dewalt_gyro_screwdriver_holder_v4 (Autodesk Fusion 360 design; units mm, degrees)
Autodesk Fusion 360 part; units mm, degrees
sketch "Sketch1" plane through (0, 0, 0) normal (0, 0, 1) x (1, 0, 0)
  line L0 (0, 0) -> (38.1, 0)
  line L1 (38.1, 0) -> (38.1, 38.1)
  line L2 (38.1, 38.1) -> (0, 38.1)
  line L3 (0, 38.1) -> (0, 0)
  dimension "d1" = 38.1
  dimension "d2" = 38.1
  constraint horizontal L0
  constraint vertical L1
  constraint horizontal L2
  constraint vertical L3
  constraint coincident L0.start L3.end
  measures "d1" distance of L0.start L2.end
  measures "d2" distance of L0.start L0.end
extrude "Extrude1" add sketch "Sketch1" along normal blind 1 makes body 1
sketch "Sketch3" plane through (0, 38.1, 0) normal (0, 1, 0) x (-1, 0, 0)
  line L0 (-38.1, 0) -> (0, 0)
  line L1 (0, 0) -> (0, 1)
  line L2 (0, 1) -> (-38.1, 1)
  line L3 (-38.1, 1) -> (-38.1, 0)
  circle A0 centre (-19.05, 13) radius 10
  line L4 (-7.05, 1) -> (-31.05, 1)
  line L5 (-31.05, 1) -> (-31.05, 13)
  line L6 (-19.05, 25) -> (-19.05, 25)
  line L7 (-7.05, 13) -> (-7.05, 1)
  arc A1 (-7.05, 13) -> (-19.05, 25) centre (-19.05, 13) ccw
  arc A2 (-19.05, 25) -> (-31.05, 13) centre (-19.05, 13) ccw
  dimension "d40" = 20
  dimension "d44" = 12
  dimension "d45" = 12
  dimension "d46" = 12
  dimension "d48" = 19.05
  dimension "d49" = 19.05
  dimension "d50" = 12
  constraint horizontal L4
  constraint vertical L5
  constraint vertical L7
  constraint coincident L2 L4.start
  constraint tangent L7 A1
  constraint tangent L5 A2
  constraint equal A1 A2
  measures "d40" diameter of A0
  measures "d44" distance of L2 A0.centre
  measures "d45" distance of A0.centre L7
  measures "d46" distance of A0.centre L5
  measures "d48" distance of L3 A0.centre
  measures "d49" distance of L1 A0.centre
  measures "d50" radius of A1
extrude "Extrude9" add sketch "Sketch3" against normal blind 46 separate body contours A0 makes body 2
extrude "Extrude2" add sketch "Sketch3" along normal blind 20 separate body contours L2 L4 L5 L7 A1 A2 | A0 makes body 3
move_body "Move1" bodies 3 to x (1, 0, 0) y (0, 1, 0) z (0, 0, 1) at (0, -32, 0)
move_body "Align1" bodies 3 to x (1, 0, 0) y (0, 1, 0) z (0, 0, 1) at (-0.0025, 2.95, -24)
move_body "Move2" bodies 3 to x (1, 0, 0) y (0, 1, 0) z (0, 0, 1) at (0, 0, 27)
move_body "Move3" bodies 3 to x (1, 0, 0) y (0, 1, 0) z (0, 0, 1) at (0, 0, 5)
move_body "Align2" bodies 3 to x (1, 0, 0) y (0, 1, 0) z (0, 0, 1) at (0, 0, -8)
fillet "Fillet1" radius 6 1 edges at (38.1, 38.1, 0.5) on bodies 1
fillet "Fillet2" radius 6 1 edges at (0, 38.1, 0.5) on bodies 1
fillet "Fillet3" radius 6 1 edges at (0, 0, 0.5) on bodies 1
fillet "Fillet4" radius 6 1 edges at (38.1, 0, 0.5) on bodies 1
sketch "Sketch4" plane through (0, 0, 1) normal (0, 0, 1) x (1, 0, 0)
  arc A0 (32.1, 0) -> (38.1, 6) centre (32.1, 6) ccw
  line L0 (38.1, 6) -> (38.1, 32.1)
  arc A1 (38.1, 32.1) -> (32.1, 38.1) centre (32.1, 32.1) ccw
  line L1 (32.1, 38.1) -> (6, 38.1)
  arc A2 (6, 38.1) -> (0, 32.1) centre (6, 32.1) ccw
  line L2 (0, 32.1) -> (0, 6)
  arc A3 (0, 6) -> (6, 0) centre (6, 6) ccw
  line L3 (6, 0) -> (32.1, 0)
  circle A4 centre (19.05, 33.1) radius 1.5
  circle A5 centre (19.05, 5) radius 1.5
  circle A6 centre (19.05, 5) radius 4
  circle A7 centre (19.05, 33.1) radius 4
  dimension "d21" = 3
  dimension "d22" = 5
  dimension "d23" = 3
  dimension "d24" = 5
  dimension "d29" = 8
  dimension "d30" = 8
  constraint concentric A5 A6
  constraint concentric A4 A7
  measures "d21" diameter of A4
  measures "d22" distance of L1 A4.centre
  measures "d23" diameter of A5
  measures "d24" distance of L3 A5.centre
  measures "d29" diameter of A6
  measures "d30" diameter of A7
combine "Combine1" operation cut target body 3 tool bodies 2
fillet "Fillet5" radius 1 1 edges at (28.3733, 29.05, 16.6162) on bodies 3
fillet "Fillet6" radius 1 1 edges at (28.3733, 9.05, 9.3838) on bodies 3
extrude "Extrude10" cut sketch "Sketch4" against normal blind 7 contours A4 bodies 1
extrude "Extrude11" cut sketch "Sketch4" against normal blind 17 contours A5 bodies 1
extrude "Extrude12" cut sketch "Sketch4" against normal blind 0.75 contours A6 bodies 1
extrude "Extrude13" cut sketch "Sketch4" against normal blind 0.75 contours A7 bodies 1
extrude "Extrude4" [suppressed]
extrude "Extrude3" [suppressed]
extrude "Extrude5" [suppressed]
extrude "Extrude6" [suppressed]
move_face "OffsetFaces1" [suppressed]
extrude "Extrude7" [suppressed]
extrude "Extrude8" [suppressed]
